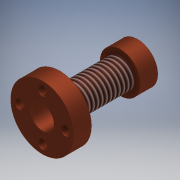
# Autodesk Inventor part: tuerca anti backlash
Saved by Autodesk Inventor 2018 (Build 220112000, 112)
## iProperties
Created: 2019-05-16
Part Number: tuerca anti backlash
Material: Generic
Document SubType Name: Modeling
Designer: JLVega003
Density: 1 g/cm^3
Appearance: Copper - Satin
Author: JLVega003
Autodesk Inventor part; units mm, degrees
ref_plane "YZ Plane" through (0, 0, 0) normal (1, 0, 0) x (0, 1, 0)
ref_plane "XZ Plane" through (0, 0, 0) normal (0, 1, 0) x (-1, 0, 0)
ref_plane "XY Plane" through (0, 0, 0) normal (0, 0, 1) x (1, 0, 0)
sketch "Sketch1" plane through (0, 0, 0) normal (0, 0, 1) x (1, 0, 0)
  line L0 (7, 33) -> (7, 27)
  line L1 (7, 27) -> (5, 27)
  line L2 (5, 27) -> (5, 6)
  line L3 (5, 6) -> (11, 6)
  line L4 (11, 6) -> (11, 0)
  line L5 (4, 33) -> (4, 0)
  line L6 (4, 33) -> (7, 33)
  line L7 (4, 0) -> (11, 0)
  line L8 (-2.2, 0) -> (13.2, 0) projected
  line L9 (0, -6.6) -> (0, 39.6) projected
  point P0 (0, 0)
  dimension "d9" = 8
  dimension "d10" = 14
  dimension "d11" = 22
  dimension "d12" = 10
  dimension "d13" = 6
  dimension "d14" = 6
  dimension "d15" = 33
  constraints: 16 end point, 4 perpendicular, 1 collinear, 1 horizontal, 1 parallel
  measures "d9" diameter of L5 L9
  measures "d10" diameter of L0 L9
  measures "d11" diameter of L4 L9
  measures "d12" diameter of L2 L9
  measures "d13" distance between parallel lines of L7 L3
  measures "d14" distance between parallel lines of L1 L6
  measures "d15" distance between parallel lines of L8 L6
revolve "Revolution2" add sketch "Sketch1" angle 360 about axis through (0, -10, 0) along (0, 1, 0)
thread "Thread2" size "M10x1.5" class "6g" standard "ISO Metric profile" full length
sketch "Sketch2" plane through (0, 6, 0) normal (0, 1, 0) x (1, 0, 0)
  circle A0 centre (0, 0) radius 8
  line L0 (-15.4, 0) -> (15.4, 0) projected
  line L1 (0, 15.4) -> (0, -15.4) projected
  point P0 (-8, 0)
  point P1 (0, -8)
  point P2 (0, 8)
  point P3 (8, 0)
  dimension "d19" = 16
  constraints: 4 point on circle, 4 point on line, 1 centre point, 1 coincident
  measures "d19" diameter of A0
hole "Hole1" at (-8, 6, 0) at (0, 6, 8) at (0, 6, -8) at (8, 6, 0) direction (0, -1, 0) diameter 3.4 depth 8 tip angle 118
body "Solid2"
